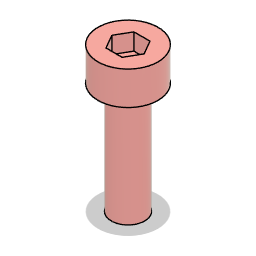
Mini_Barrett_Hand (Autodesk Fusion 360 archive; units mm, degrees)
design "M3*10"
Autodesk Fusion 360 part; units mm, degrees
sketch "Sketch1" plane through (0, 0, 0) normal (0, 1, 0) x (1, 0, 0)
  circle A0 centre (0, 0) radius 1.5
  dimension "d1" = 3
  constraint coincident A0.centre origin
  measures "d1" diameter of A0
extrude "Extrude1" add sketch "Sketch1" along normal blind 10
sketch "Sketch2" plane through (0, 10, 0) normal (0, 1, 0) x (-1, 0, 0)
  circle A0 centre (0, 0) radius 1.5
  circle A1 centre (0, 0) radius 2.7
  dimension "d4" = 5.4
  constraint coincident A0.centre A1.centre
  measures "d4" diameter of A1
extrude "Extrude2" add sketch "Sketch2" along normal blind 3 contours A0 | A1
sketch "Sketch3" plane through (0, 13, 0) normal (0, 1, 0) x (-1, 0, 0)
  circle A0 centre (0, 0) radius 2.7
  line L0 (-0.725, 1.2557) -> (-1.45, 0)
  line L1 (-1.45, 0) -> (-0.725, -1.2557)
  line L2 (-0.725, -1.2557) -> (0.725, -1.2557)
  line L3 (0.725, -1.2557) -> (1.45, 0)
  line L4 (1.45, 0) -> (0.725, 1.2557)
  line L5 (0.725, 1.2557) -> (-0.725, 1.2557)
  dimension "d7" = 1.45
  constraint coincident A0.centre origin
  constraint horizontal L5
  measures "d7" distance of L0.start A0.centre
extrude "Extrude3" cut sketch "Sketch3" against normal blind 1.5 contours L0 L1 L2 L3 L4 L5
equation "d7 = ( 2.9 / 2 ) * 1 mm"

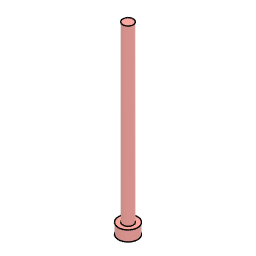
design "M3*50"
Autodesk Fusion 360 part; units mm, degrees
sketch "Sketch1" plane through (0, 0, 0) normal (0, 1, 0) x (1, 0, 0)
  circle A0 centre (0, 0) radius 2.75
  dimension "d1" = 5.5
  constraint coincident A0.centre origin
  measures "d1" diameter of A0
extrude "Extrude1" add sketch "Sketch1" along normal blind 3
sketch "Sketch2" plane through (0, 3, 0) normal (0, 1, 0) x (-1, 0, 0)
  circle A0 centre (0, 0) radius 2.75
  circle A1 centre (0, 0) radius 1.5
  dimension "d4" = 3
  constraint concentric A0 A1
  measures "d4" diameter of A1
extrude "Extrude2" add sketch "Sketch2" along normal blind 50 contours A1
sketch "Sketch3" plane through (0, 0, 0) normal (0, -1, 0) x (1, 0, 0)
  circle A0 centre (0, 0) radius 2.75
  circle A1 centre (0, 0) radius 1.25
  line L0 (0, 0) -> (0, 1.25) construction
  line L1 (0, 0) -> (-1.0825, 0.625) construction
  line L2 (0, 0) -> (-1.0825, -0.625) construction
  line L3 (0, 0) -> (0, -1.25) construction
  line L4 (0, 0) -> (1.0825, -0.625) construction
  line L5 (0, 0) -> (1.0825, 0.625) construction
  line L6 (0, 1.25) -> (1.0825, 0.625)
  line L7 (1.0825, 0.625) -> (1.0825, -0.625)
  line L8 (1.0825, -0.625) -> (0, -1.25)
  line L9 (0, -1.25) -> (-1.0825, -0.625)
  line L10 (-1.0825, -0.625) -> (-1.0825, 0.625)
  line L11 (-1.0825, 0.625) -> (0, 1.25)
  dimension "d7" = 2.5
  dimension "d9" = 360
  constraint concentric A0 A1
  constraint coincident A0.centre A1.centre
  constraint coincident A1 L0.end
  constraint vertical L0
  measures "d7" diameter of A1
extrude "Extrude3" cut sketch "Sketch3" against normal blind 1.8 contours L6 L7 L8 L9 L10 L11

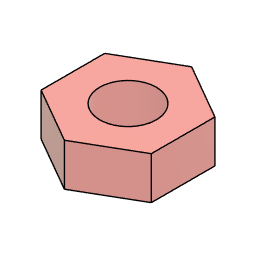
design "M2 nut"
Autodesk Fusion 360 part; units mm, degrees
sketch "Sketch1" plane through (0, 0, 0) normal (0, 1, 0) x (1, 0, 0)
  circle A0 centre (0, 0) radius 1.95 construction
  line L0 (0, 0) -> (-1.95, 0) construction
  line L1 (-1.95, 3) -> (-1.95, -3)
  line L2 (-3.5731, -0.1887) -> (1.6231, -3.1887)
  line L3 (-1.6231, -3.1887) -> (3.5731, -0.1887)
  line L4 (1.95, -3) -> (1.95, 3)
  line L5 (3.5731, 0.1887) -> (-1.6231, 3.1887)
  line L6 (1.6231, 3.1887) -> (-3.5731, 0.1887)
  circle A1 centre (0, 0) radius 1
  dimension "d1" = 3.9
  dimension "d2" = 6
  dimension "d4" = 360
  dimension "d5" = 2
  constraint coincident A0.centre L0.start
  constraint coincident A0 L0.end
  constraint horizontal L0
  constraint vertical L1
  constraint tangent A0 L1
  constraint concentric A0 A1
  measures "d1" diameter of A0
  measures "d2" distance of L1.start L1.end
  measures "d5" diameter of A1
extrude "Extrude1" add sketch "Sketch1" along normal blind 1.5

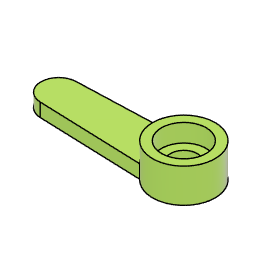
design "mounts"
Autodesk Fusion 360 part; units mm, degrees
sketch "Sketch1" plane through (0, 0, 0) normal (0, 1, 0) x (1, 0, 0)
  circle A0 centre (0, 0) radius 3.5
  line L0 (0, 0) -> (-16, 0) construction
  line L1 (-16, 0) -> (-16, -0.2121) construction
  line L2 (-16, 0) -> (-14, 0) construction
  circle A1 centre (-14, 0) radius 2
  circle A2 centre (0, 0) radius 2.5 construction
  line L3 (-15.3753, 1.9521) -> (4.4202, 2.6596)
  line L4 (-15.3753, -1.9521) -> (4.4202, -2.6596)
  dimension "d1" = 7
  dimension "d2" = 16
  dimension "d3" = 2
  dimension "d4" = 4
  dimension "d5" = 5
  constraint coincident A0.centre L0.start
  constraint horizontal L0
  constraint perpendicular L0 L1
  constraint perpendicular L1 L2
  constraint coincident L2.end A1.centre
  constraint tangent A1 L3
  constraint tangent A2 L3
  constraint symmetric L0 L3.start L4.start
  constraint symmetric L0 L3.end L4.end
  measures "d1" diameter of A0
  measures "d2" distance of A0.centre L0.end
  measures "d3" distance of L0.end L2.end
  measures "d4" diameter of A1
  measures "d5" diameter of A2
extrude "Extrude1" add sketch "Sketch1" along normal blind 1.5
sketch "Sketch2" plane through (0, 1.5, 0) normal (0, 1, 0) x (-1, 0, 0)
  arc A0 (14.0714, -1.9987) -> (14.0714, 1.9987) centre (14, 0) ccw
  line L0 (14.0714, 1.9987) -> (2.5372, 2.4109)
  arc A1 (2.5372, 2.4109) -> (2.5372, -2.4109) centre (0, 0) ccw
  line L1 (2.5372, -2.4109) -> (14.0714, -1.9987)
  circle A2 centre (0, 0) radius 3.5
  constraint concentric A1 A2
  constraint coincident A1.end A2
extrude "Extrude2" add sketch "Sketch2" along normal blind 2.3 contours A1 A2
hole "Hole1" at (0, 3.8, 0) direction (0, -1, 0) diameter 5 depth 2 tip angle 180
sketch "Sketch3" plane through (0, 0, 0) normal (0, -1, 0) x (1, 0, 0)
  arc A0 (-14.0714, 1.9987) -> (-14.0714, -1.9987) centre (-14, 0) ccw
  line L0 (-14.0714, -1.9987) -> (-2.5372, -2.4109)
  arc A1 (-2.5372, -2.4109) -> (-2.5372, 2.4109) centre (0, 0) ccw
  line L1 (-2.5372, 2.4109) -> (-14.0714, 1.9987)
  circle A2 centre (0, 0) radius 2.5
  dimension "d13" = 5
  constraint concentric A1 A2
  measures "d13" diameter of A2
extrude "Extrude3" cut sketch "Sketch3" against normal blind 1 contours A2
hole "Hole2" at (0, 1.8, 0) direction (0, -1, 0) diameter 3 depth 2 tip angle 180
equation "d2 = 19.5 mm - 3.5 mm"

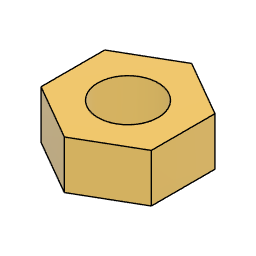
design "NutM3"
Autodesk Fusion 360 part; units mm, degrees
sketch "Sketch1" plane through (0, 0, 0) normal (0, 1, 0) x (1, 0, 0)
  circle A0 centre (0, 0) radius 2.75
  line L0 (0, 0) -> (-2.75, 0) construction
  line L1 (-2.75, 2.7896) -> (-2.75, -3.2287)
  line L2 (-3.7909, -0.9868) -> (1.4211, -3.9959)
  line L3 (-1.0409, -3.7764) -> (4.1711, -0.7672)
  line L4 (2.75, -2.7896) -> (2.75, 3.2287)
  line L5 (3.7909, 0.9868) -> (-1.4211, 3.9959)
  line L6 (1.0409, 3.7764) -> (-4.1711, 0.7672)
  circle A1 centre (0, 0) radius 1.5
  dimension "d1" = 5.5
  dimension "d3" = 360
  dimension "d6" = 3
  constraint coincident A0.centre L0.start
  constraint coincident A0 L0.end
  constraint horizontal L0
  constraint vertical L1
  constraint tangent A0 L1
  constraint concentric A0 A1
  measures "d1" diameter of A0
  measures "d6" diameter of A1
extrude "Extrude1" add sketch "Sketch1" along normal blind 2.4

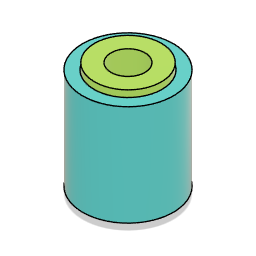
design "bush"
Autodesk Fusion 360 part; units mm, degrees
sketch "Sketch1" plane through (0, 0, 0) normal (0, 1, 0) x (1, 0, 0) in component "outer"
  circle A0 centre (0, 0) radius 4
  dimension "d1" = 8
  constraint coincident A0.centre origin
  measures "d1" diameter of A0
extrude "Extrude1" add sketch "Sketch1" along normal blind 8.9 makes body 1 in component "outer"
sketch "Sketch2" plane through (0, 0, 0) normal (0, -1, 0) x (1, 0, 0) in component "outer"
  circle A0 centre (0, 0) radius 4
  circle A1 centre (0, 0) radius 3
  dimension "d4" = 6
  constraint concentric A0 A1
  measures "d4" diameter of A1
extrude "Extrude2" cut sketch "Sketch2" against normal blind 12 contours A1 bodies 1 in component "outer"
sketch "Sketch1 (2)" plane through (0, 0, 0) normal (0, 1, 0) x (1, 0, 0) in component "inner"
  circle A0 centre (0, 0) radius 2.95
  dimension "d7" = 5.9
  constraint coincident A0.centre origin
  measures "d7" diameter of A0
extrude "Extrude1'" add sketch "Sketch1 (2)" along normal blind 10 separate body makes body 2 in component "inner"
sketch "Sketch2 (2)" plane through (0, 10, 0) normal (0, 1, 0) x (-1, 0, 0) in component "inner"
  circle A0 centre (0, 0) radius 2.95
  circle A1 centre (0, 0) radius 1.5
  dimension "d10" = 3
  constraint concentric A0 A1
  measures "d10" diameter of A1
extrude "Extrude2'" cut sketch "Sketch2 (2)" against normal blind 11 contours A1 bodies 2 in component "inner"
component "outer" placed x (1, 0, 0) y (0, 1, 0) z (0, 0, 1) at (0, 0, 0)
component "inner" placed x (1, 0, 0) y (0, 1, 0) z (0, 0, 1) at (0, -0.55, 0)

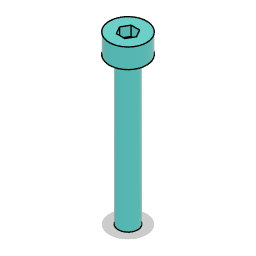
design "M2*15"
Autodesk Fusion 360 part; units mm, degrees
sketch "Sketch1" plane through (0, 0, 0) normal (0, 1, 0) x (1, 0, 0)
  circle A0 centre (0, 0) radius 1
  dimension "d1" = 2
  constraint coincident A0.centre origin
  measures "d1" diameter of A0
extrude "Extrude1" add sketch "Sketch1" along normal blind 15
sketch "Sketch2" plane through (0, 15, 0) normal (0, 1, 0) x (-1, 0, 0)
  circle A0 centre (0, 0) radius 1
  circle A1 centre (0, 0) radius 1.9
  dimension "d4" = 3.8
  constraint coincident A0.centre A1.centre
  measures "d4" diameter of A1
extrude "Extrude2" add sketch "Sketch2" along normal blind 2 contours A0 | A1
sketch "Sketch3" plane through (0, 17, 0) normal (0, 1, 0) x (-1, 0, 0)
  circle A0 centre (0, 0) radius 1.9
  line L0 (-0.866, 0) -> (-0.433, -0.75)
  line L1 (-0.433, -0.75) -> (0.433, -0.75)
  line L2 (0.433, -0.75) -> (0.866, 0)
  line L3 (0.866, 0) -> (0.433, 0.75)
  line L4 (0.433, 0.75) -> (-0.433, 0.75)
  line L5 (-0.433, 0.75) -> (-0.866, 0)
  dimension "d7" = 0.75
  constraint coincident A0.centre origin
  constraint horizontal L4
  measures "d7" distance of A0.centre L5
extrude "Extrude3" cut sketch "Sketch3" against normal blind 1 contours L0 L1 L2 L3 L4 L5
equation "d7 = ( 1.5 / 2 ) * 1 mm"
